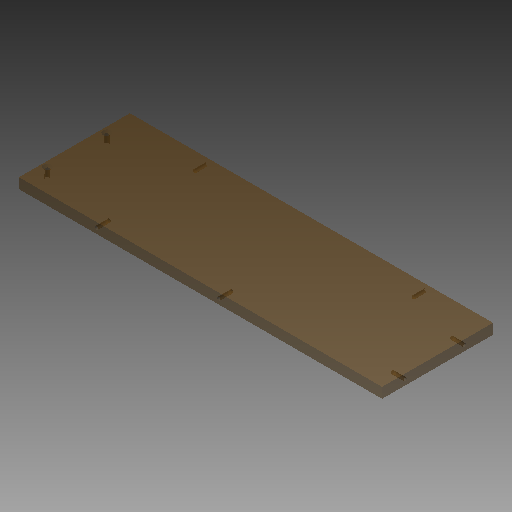
# Autodesk Inventor part: Wand4
Saved by Autodesk Inventor 2018 (Build 220112000, 112)
## iProperties
Created: 2013-02-21
Part Number: Wand4
Material: Polycarbonate, Smoke
Document SubType Name: Modeling
Designer: Neef
Mass: 232.406 g
Surface Area: 542.98 cm^2
Volume: 193.672 cm^3
Density: 1.2 g/cm^3
Appearance: Polycarbonate - Smoked
Author: Neef
Autodesk Inventor part; units mm, degrees
ref_plane "YZ Plane" through (0, 0, 0) normal (1, 0, 0) x (0, 1, 0)
ref_plane "XZ Plane" through (0, 0, 0) normal (0, 1, 0) x (-1, 0, 0)
ref_plane "XY Plane" through (0, 0, 0) normal (0, 0, 1) x (1, 0, 0)
sketch "Skizze1" plane through (0, 0, 0) normal (0, 0, 1) x (1, 0, 0)
  line L0 (-140.75, 43) -> (140.75, 43)
  line L1 (140.75, 43) -> (140.75, -43)
  line L2 (140.75, -43) -> (-140.75, -43)
  line L3 (-140.75, -43) -> (-140.75, 43)
  line L4 (0, 60.2) -> (0, -60.2) projected
  line L5 (-197.05, 0) -> (197.05, 0) projected
  point P0 (0, 0)
  point P1 (0, 43)
  point P2 (-140.75, 0)
  dimension "d0" = 281.5
  dimension "d1" = 86
  constraints: 8 end point, 2 midpoint, 2 parallel, 2 point on line, 1 horizontal, 1 perpendicular
  measures "d0" distance of L0.start L0.end
  measures "d1" distance of L2.end L0.start
extrude "Extrusion1" add sketch "Skizze1" along normal blind 8
sketch "Skizze2" plane through (-140.75, 43, 0) normal (0, 1, 0) x (1, 0, 0)
  circle A0 centre (285.5, 42) radius 3.1 projected
  circle A1 centre (60, -4) radius 3.1 projected
  circle A2 centre (229.5, -4) radius 3.1 projected
  circle A3 centre (4, 42) radius 3.1 projected
  circle A4 centre (285.5, 142) radius 3.1 projected
  circle A5 centre (4, 142) radius 3.1 projected
  circle A6 centre (229.5, 188) radius 3.1 projected
  circle A7 centre (60, 188) radius 3.1 projected
  line L0 (0, -8) -> (0, 192) projected
  line L1 (0, -8) -> (289.5, -8) projected
  line L2 (289.5, -8) -> (289.5, 69) projected
  line L3 (289.5, 69) -> (341.5, 69) projected
  line L4 (341.5, 69) -> (341.5, 115) projected
  line L5 (289.5, 115) -> (341.5, 115) projected
  line L6 (289.5, 192) -> (289.5, 115) projected
  line L7 (0, 192) -> (289.5, 192) projected
  point P0 (140.75, 0)
  constraints: 2 coincident
hole "Bohrung1" at (-80.75, 43, 4) at (88.75, 43, 4) direction (0, -1, 0) diameter 2.459 depth 10 tip angle 118 thread size "M3x0.5" class "6H" standard "ISO Metric profile"
sketch "Skizze3" plane through (140.75, -43, 0) normal (1, 0, 0) x (0, 0, -1)
  circle A0 centre (-4, 18) radius 3.15 projected
  circle A1 centre (-4, 64) radius 3.15 projected
  line L0 (69, 18.5) -> (69, 86) projected
  line L1 (-8, 86) -> (69, 86) projected
  line L2 (-8, -4) -> (-8, 86) projected
  line L3 (87.2303, -4) -> (-8, -4) projected
  arc A2 (69, 18.5) -> (87.2303, -4) centre (92, 18.5) ccw projected
  point P0 (0, 43)
  constraints: 2 coincident
hole "Bohrung2" at (140.75, -25, 4) at (140.75, 21, 4) direction (-1, 0, 0) diameter 2.459 depth 10 tip angle 118 thread size "M3x0.5" class "6H" standard "ISO Metric profile"
sketch "Skizze4" plane through (0, 0, 8) normal (0, 0, 1) x (1, 0, 0)
  line L0 (-140.75, 43) -> (140.75, 43) projected
  line L1 (-140.75, -43) -> (-140.75, 43) projected
  line L2 (140.75, -43) -> (-140.75, -43) projected
  point P0 (0, 0)
  point P1 (-136.75, 21)
  point P2 (-136.75, -25)
  dimension "d18" = 4
  dimension "d19" = 22
  dimension "d20" = 4
  dimension "d21" = 18
  measures "d18" distance from line of L1 point (-136.75, 21)
  measures "d19" distance from line of L0 point (-136.75, 21)
  measures "d20" distance from line of L1 point (-136.75, -25)
  measures "d21" distance from line of point (-136.75, -25) L2
hole "Bohrung3" at (-136.75, 21, 8) at (-136.75, -25, 8) direction (0, 0, -1) diameter 3.2 end through all countersink diameter 6.2 countersink angle 90
sketch "Skizze5" plane through (-140.75, -43, 0) normal (0, -1, 0) x (1, 0, 0)
  circle A0 centre (60, 4) radius 3.1 projected
  circle A1 centre (155, 4) radius 3.1 projected
  point P0 (140.75, 0)
  constraints: 2 coincident
hole "Bohrung4" at (-80.75, -43, 4) at (14.25, -43, 4) direction (0, 1, 0) diameter 2.459 depth 10 tip angle 118 thread size "M3x0.5" class "6H" standard "ISO Metric profile"
equation "\"d20\" = d18"
